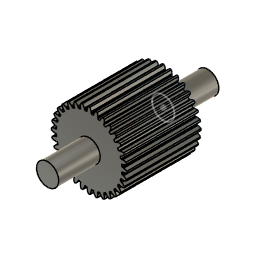
New_Spur_and_Rod v4 (Autodesk Fusion 360 design; units mm, degrees)
description: Spur Gear; Module: 0.750000; Number of Teeth: 32; Pressure Angle: 20.000000; Root Fillet Radius: 0.032000; Clearance: 0.000000; Gear Thickness: 2.500000; Hole Diameter: 0.750000;
Autodesk Fusion 360 part; units mm, degrees
sketch "Sketch1" plane through (0, 0, 0) normal (0, 1, 0) x (1, 0, 0) in component "Spur Gear (32 teeth)"
  arc A0 (10.9657, -1.4605) -> (11.0399, -0.7069) centre (0, 0) ccw
  line L0 (11.0399, -0.7069) -> (11.2693, -0.7216)
  spline S0 degree 3 poles (11.2693, -0.7216) (11.3119, -0.7221) (11.4405, -0.7189) (11.6548, -0.6748) knots 0 0 0 0 1 1 1 1
  spline S1 degree 3 poles (11.6548, -0.6748) (11.911, -0.6218) (12.2826, -0.5105) (12.7477, -0.2784) knots 0 0 0 0 1 1 1 1
  arc A1 (12.7477, -0.2784) -> (12.7477, 0.2784) centre (0, 0) ccw
  spline S2 degree 3 poles (12.7477, 0.2784) (12.2826, 0.5105) (11.911, 0.6218) (11.6548, 0.6748) knots 0 0 0 0 1 1 1 1
  spline S3 degree 3 poles (11.6548, 0.6748) (11.4405, 0.7189) (11.3119, 0.7221) (11.2693, 0.7216) knots 0 0 0 0 1 1 1 1
  line L1 (11.2693, 0.7216) -> (11.0399, 0.7069)
  arc A2 (11.0399, 0.7069) -> (10.9657, 1.4605) centre (0, 0) ccw
  line L2 (10.9657, 1.4605) -> (11.1935, 1.4908)
  spline S4 degree 3 poles (11.1935, 1.4908) (11.2354, 1.4987) (11.3609, 1.5268) (11.5625, 1.6119) knots 0 0 0 0 1 1 1 1
  spline S5 degree 3 poles (11.5625, 1.6119) (11.8034, 1.7139) (12.1462, 1.8956) (12.5571, 2.2139) knots 0 0 0 0 1 1 1 1
  arc A3 (12.5571, 2.2139) -> (12.4485, 2.76) centre (0, 0) ccw
  spline S6 degree 3 poles (12.4485, 2.76) (11.947, 2.8969) (11.5608, 2.9336) (11.2992, 2.9356) knots 0 0 0 0 1 1 1 1
  spline S7 degree 3 poles (11.2992, 2.9356) (11.0804, 2.937) (10.9537, 2.915) (10.912, 2.9063) knots 0 0 0 0 1 1 1 1
  line L3 (10.912, 2.9063) -> (10.6899, 2.8471)
  arc A4 (10.6899, 2.8471) -> (10.47, 3.5717) centre (0, 0) ccw
  line L4 (10.47, 3.5717) -> (10.6876, 3.6459)
  spline S8 degree 3 poles (10.6876, 3.6459) (10.7272, 3.6618) (10.8448, 3.7139) (11.0259, 3.8367) knots 0 0 0 0 1 1 1 1
  spline S9 degree 3 poles (11.0259, 3.8367) (11.2423, 3.9837) (11.543, 4.2287) (11.8839, 4.6211) knots 0 0 0 0 1 1 1 1
  arc A5 (11.8839, 4.6211) -> (11.6708, 5.1356) centre (0, 0) ccw
  spline S10 degree 3 poles (11.6708, 5.1356) (11.1523, 5.1719) (10.7664, 5.1326) (10.5094, 5.0835) knots 0 0 0 0 1 1 1 1
  spline S11 degree 3 poles (10.5094, 5.0835) (10.2945, 5.0423) (10.1746, 4.996) (10.1353, 4.9792) knots 0 0 0 0 1 1 1 1
  line L5 (10.1353, 4.9792) -> (9.929, 4.8779)
  arc A6 (9.929, 4.8779) -> (9.5721, 5.5457) centre (0, 0) ccw
  line L6 (9.5721, 5.5457) -> (9.771, 5.6609)
  spline S12 degree 3 poles (9.771, 5.6609) (9.8067, 5.6842) (9.9118, 5.7583) (10.0655, 5.914) knots 0 0 0 0 1 1 1 1
  spline S13 degree 3 poles (10.0655, 5.914) (10.2491, 6.1004) (10.4962, 6.3994) (10.754, 6.8508) knots 0 0 0 0 1 1 1 1
  arc A7 (10.754, 6.8508) -> (10.4447, 7.3137) centre (0, 0) ccw
  spline S14 degree 3 poles (10.4447, 7.3137) (9.929, 7.2483) (9.5582, 7.1344) (9.3157, 7.0361) knots 0 0 0 0 1 1 1 1
  spline S15 degree 3 poles (9.3157, 7.0361) (9.113, 6.9538) (9.0044, 6.8849) (8.9692, 6.8609) knots 0 0 0 0 1 1 1 1
  line L7 (8.9692, 6.8609) -> (8.7866, 6.7212)
  arc A8 (8.7866, 6.7212) -> (8.3062, 7.3065) centre (0, 0) ccw
  line L8 (8.3062, 7.3065) -> (8.4788, 7.4584)
  spline S16 degree 3 poles (8.4788, 7.4584) (8.5093, 7.4882) (8.598, 7.5813) (8.7184, 7.7641) knots 0 0 0 0 1 1 1 1
  spline S17 degree 3 poles (8.7184, 7.7641) (8.862, 7.9827) (9.046, 8.3242) (9.2109, 8.8171) knots 0 0 0 0 1 1 1 1
  arc A9 (9.2109, 8.8171) -> (8.8171, 9.2109) centre (0, 0) ccw
  spline S18 degree 3 poles (8.8171, 9.2109) (8.3242, 9.046) (7.9827, 8.862) (7.7641, 8.7184) knots 0 0 0 0 1 1 1 1
  spline S19 degree 3 poles (7.7641, 8.7184) (7.5813, 8.598) (7.4882, 8.5093) (7.4584, 8.4788) knots 0 0 0 0 1 1 1 1
  line L9 (7.4584, 8.4788) -> (7.3065, 8.3062)
  arc A10 (7.3065, 8.3062) -> (6.7212, 8.7866) centre (0, 0) ccw
  line L10 (6.7212, 8.7866) -> (6.8609, 8.9692)
  spline S20 degree 3 poles (6.8609, 8.9692) (6.8849, 9.0044) (6.9538, 9.113) (7.0361, 9.3157) knots 0 0 0 0 1 1 1 1
  spline S21 degree 3 poles (7.0361, 9.3157) (7.1344, 9.5582) (7.2483, 9.929) (7.3137, 10.4447) knots 0 0 0 0 1 1 1 1
  arc A11 (7.3137, 10.4447) -> (6.8508, 10.754) centre (0, 0) ccw
  spline S22 degree 3 poles (6.8508, 10.754) (6.3994, 10.4962) (6.1004, 10.2491) (5.914, 10.0655) knots 0 0 0 0 1 1 1 1
  spline S23 degree 3 poles (5.914, 10.0655) (5.7583, 9.9118) (5.6842, 9.8067) (5.6609, 9.771) knots 0 0 0 0 1 1 1 1
  line L11 (5.6609, 9.771) -> (5.5457, 9.5721)
  arc A12 (5.5457, 9.5721) -> (4.8779, 9.929) centre (0, 0) ccw
  line L12 (4.8779, 9.929) -> (4.9792, 10.1353)
  spline S24 degree 3 poles (4.9792, 10.1353) (4.996, 10.1746) (5.0423, 10.2945) (5.0835, 10.5094) knots 0 0 0 0 1 1 1 1
  spline S25 degree 3 poles (5.0835, 10.5094) (5.1326, 10.7664) (5.1719, 11.1523) (5.1356, 11.6708) knots 0 0 0 0 1 1 1 1
  arc A13 (5.1356, 11.6708) -> (4.6211, 11.8839) centre (0, 0) ccw
  spline S26 degree 3 poles (4.6211, 11.8839) (4.2287, 11.543) (3.9837, 11.2423) (3.8367, 11.0259) knots 0 0 0 0 1 1 1 1
  spline S27 degree 3 poles (3.8367, 11.0259) (3.7139, 10.8448) (3.6618, 10.7272) (3.6459, 10.6876) knots 0 0 0 0 1 1 1 1
  line L13 (3.6459, 10.6876) -> (3.5717, 10.47)
  arc A14 (3.5717, 10.47) -> (2.8471, 10.6899) centre (0, 0) ccw
  line L14 (2.8471, 10.6899) -> (2.9063, 10.912)
  spline S28 degree 3 poles (2.9063, 10.912) (2.915, 10.9537) (2.937, 11.0804) (2.9356, 11.2992) knots 0 0 0 0 1 1 1 1
  spline S29 degree 3 poles (2.9356, 11.2992) (2.9336, 11.5608) (2.8969, 11.947) (2.76, 12.4485) knots 0 0 0 0 1 1 1 1
  arc A15 (2.76, 12.4485) -> (2.2139, 12.5571) centre (0, 0) ccw
  spline S30 degree 3 poles (2.2139, 12.5571) (1.8956, 12.1462) (1.7139, 11.8034) (1.6119, 11.5625) knots 0 0 0 0 1 1 1 1
  spline S31 degree 3 poles (1.6119, 11.5625) (1.5268, 11.3609) (1.4987, 11.2354) (1.4908, 11.1935) knots 0 0 0 0 1 1 1 1
  line L15 (1.4908, 11.1935) -> (1.4605, 10.9657)
  arc A16 (1.4605, 10.9657) -> (0.7069, 11.0399) centre (0, 0) ccw
  line L16 (0.7069, 11.0399) -> (0.7216, 11.2693)
  spline S32 degree 3 poles (0.7216, 11.2693) (0.7221, 11.3119) (0.7189, 11.4405) (0.6748, 11.6548) knots 0 0 0 0 1 1 1 1
  spline S33 degree 3 poles (0.6748, 11.6548) (0.6218, 11.911) (0.5105, 12.2826) (0.2784, 12.7477) knots 0 0 0 0 1 1 1 1
  arc A17 (0.2784, 12.7477) -> (-0.2784, 12.7477) centre (0, 0) ccw
  spline S34 degree 3 poles (-0.2784, 12.7477) (-0.5105, 12.2826) (-0.6218, 11.911) (-0.6748, 11.6548) knots 0 0 0 0 1 1 1 1
  spline S35 degree 3 poles (-0.6748, 11.6548) (-0.7189, 11.4405) (-0.7221, 11.3119) (-0.7216, 11.2693) knots 0 0 0 0 1 1 1 1
  line L17 (-0.7216, 11.2693) -> (-0.7069, 11.0399)
  arc A18 (-0.7069, 11.0399) -> (-1.4605, 10.9657) centre (0, 0) ccw
  line L18 (-1.4605, 10.9657) -> (-1.4908, 11.1935)
  spline S36 degree 3 poles (-1.4908, 11.1935) (-1.4987, 11.2354) (-1.5268, 11.3609) (-1.6119, 11.5625) knots 0 0 0 0 1 1 1 1
  spline S37 degree 3 poles (-1.6119, 11.5625) (-1.7139, 11.8034) (-1.8956, 12.1462) (-2.2139, 12.5571) knots 0 0 0 0 1 1 1 1
  arc A19 (-2.2139, 12.5571) -> (-2.76, 12.4485) centre (0, 0) ccw
  spline S38 degree 3 poles (-2.76, 12.4485) (-2.8969, 11.947) (-2.9336, 11.5608) (-2.9356, 11.2992) knots 0 0 0 0 1 1 1 1
  spline S39 degree 3 poles (-2.9356, 11.2992) (-2.937, 11.0804) (-2.915, 10.9537) (-2.9063, 10.912) knots 0 0 0 0 1 1 1 1
  line L19 (-2.9063, 10.912) -> (-2.8471, 10.6899)
  arc A20 (-2.8471, 10.6899) -> (-3.5717, 10.47) centre (0, 0) ccw
  line L20 (-3.5717, 10.47) -> (-3.6459, 10.6876)
  spline S40 degree 3 poles (-3.6459, 10.6876) (-3.6618, 10.7272) (-3.7139, 10.8448) (-3.8367, 11.0259) knots 0 0 0 0 1 1 1 1
  spline S41 degree 3 poles (-3.8367, 11.0259) (-3.9837, 11.2423) (-4.2287, 11.543) (-4.6211, 11.8839) knots 0 0 0 0 1 1 1 1
  arc A21 (-4.6211, 11.8839) -> (-5.1356, 11.6708) centre (0, 0) ccw
  spline S42 degree 3 poles (-5.1356, 11.6708) (-5.1719, 11.1523) (-5.1326, 10.7664) (-5.0835, 10.5094) knots 0 0 0 0 1 1 1 1
  spline S43 degree 3 poles (-5.0835, 10.5094) (-5.0423, 10.2945) (-4.996, 10.1746) (-4.9792, 10.1353) knots 0 0 0 0 1 1 1 1
  line L21 (-4.9792, 10.1353) -> (-4.8779, 9.929)
  arc A22 (-4.8779, 9.929) -> (-5.5457, 9.5721) centre (0, 0) ccw
  line L22 (-5.5457, 9.5721) -> (-5.6609, 9.771)
  spline S44 degree 3 poles (-5.6609, 9.771) (-5.6842, 9.8067) (-5.7583, 9.9118) (-5.914, 10.0655) knots 0 0 0 0 1 1 1 1
  spline S45 degree 3 poles (-5.914, 10.0655) (-6.1004, 10.2491) (-6.3994, 10.4962) (-6.8508, 10.754) knots 0 0 0 0 1 1 1 1
  arc A23 (-6.8508, 10.754) -> (-7.3137, 10.4447) centre (0, 0) ccw
  spline S46 degree 3 poles (-7.3137, 10.4447) (-7.2483, 9.929) (-7.1344, 9.5582) (-7.0361, 9.3157) knots 0 0 0 0 1 1 1 1
  spline S47 degree 3 poles (-7.0361, 9.3157) (-6.9538, 9.113) (-6.8849, 9.0044) (-6.8609, 8.9692) knots 0 0 0 0 1 1 1 1
  line L23 (-6.8609, 8.9692) -> (-6.7212, 8.7866)
  arc A24 (-6.7212, 8.7866) -> (-7.3065, 8.3062) centre (0, 0) ccw
  line L24 (-7.3065, 8.3062) -> (-7.4584, 8.4788)
  spline S48 degree 3 poles (-7.4584, 8.4788) (-7.4882, 8.5093) (-7.5813, 8.598) (-7.7641, 8.7184) knots 0 0 0 0 1 1 1 1
  spline S49 degree 3 poles (-7.7641, 8.7184) (-7.9827, 8.862) (-8.3242, 9.046) (-8.8171, 9.2109) knots 0 0 0 0 1 1 1 1
  arc A25 (-8.8171, 9.2109) -> (-9.2109, 8.8171) centre (0, 0) ccw
  spline S50 degree 3 poles (-9.2109, 8.8171) (-9.046, 8.3242) (-8.862, 7.9827) (-8.7184, 7.7641) knots 0 0 0 0 1 1 1 1
  spline S51 degree 3 poles (-8.7184, 7.7641) (-8.598, 7.5813) (-8.5093, 7.4882) (-8.4788, 7.4584) knots 0 0 0 0 1 1 1 1
  line L25 (-8.4788, 7.4584) -> (-8.3062, 7.3065)
  arc A26 (-8.3062, 7.3065) -> (-8.7866, 6.7212) centre (0, 0) ccw
  line L26 (-8.7866, 6.7212) -> (-8.9692, 6.8609)
  spline S52 degree 3 poles (-8.9692, 6.8609) (-9.0044, 6.8849) (-9.113, 6.9538) (-9.3157, 7.0361) knots 0 0 0 0 1 1 1 1
  spline S53 degree 3 poles (-9.3157, 7.0361) (-9.5582, 7.1344) (-9.929, 7.2483) (-10.4447, 7.3137) knots 0 0 0 0 1 1 1 1
  arc A27 (-10.4447, 7.3137) -> (-10.754, 6.8508) centre (0, 0) ccw
  spline S54 degree 3 poles (-10.754, 6.8508) (-10.4962, 6.3994) (-10.2491, 6.1004) (-10.0655, 5.914) knots 0 0 0 0 1 1 1 1
  spline S55 degree 3 poles (-10.0655, 5.914) (-9.9118, 5.7583) (-9.8067, 5.6842) (-9.771, 5.6609) knots 0 0 0 0 1 1 1 1
  line L27 (-9.771, 5.6609) -> (-9.5721, 5.5457)
  arc A28 (-9.5721, 5.5457) -> (-9.929, 4.8779) centre (0, 0) ccw
  line L28 (-9.929, 4.8779) -> (-10.1353, 4.9792)
  spline S56 degree 3 poles (-10.1353, 4.9792) (-10.1746, 4.996) (-10.2945, 5.0423) (-10.5094, 5.0835) knots 0 0 0 0 1 1 1 1
  spline S57 degree 3 poles (-10.5094, 5.0835) (-10.7664, 5.1326) (-11.1523, 5.1719) (-11.6708, 5.1356) knots 0 0 0 0 1 1 1 1
  arc A29 (-11.6708, 5.1356) -> (-11.8839, 4.6211) centre (0, 0) ccw
  spline S58 degree 3 poles (-11.8839, 4.6211) (-11.543, 4.2287) (-11.2423, 3.9837) (-11.0259, 3.8367) knots 0 0 0 0 1 1 1 1
  spline S59 degree 3 poles (-11.0259, 3.8367) (-10.8448, 3.7139) (-10.7272, 3.6618) (-10.6876, 3.6459) knots 0 0 0 0 1 1 1 1
  line L29 (-10.6876, 3.6459) -> (-10.47, 3.5717)
  arc A30 (-10.47, 3.5717) -> (-10.6899, 2.8471) centre (0, 0) ccw
  line L30 (-10.6899, 2.8471) -> (-10.912, 2.9063)
  spline S60 degree 3 poles (-10.912, 2.9063) (-10.9537, 2.915) (-11.0804, 2.937) (-11.2992, 2.9356) knots 0 0 0 0 1 1 1 1
  spline S61 degree 3 poles (-11.2992, 2.9356) (-11.5608, 2.9336) (-11.947, 2.8969) (-12.4485, 2.76) knots 0 0 0 0 1 1 1 1
  arc A31 (-12.4485, 2.76) -> (-12.5571, 2.2139) centre (0, 0) ccw
  spline S62 degree 3 poles (-12.5571, 2.2139) (-12.1462, 1.8956) (-11.8034, 1.7139) (-11.5625, 1.6119) knots 0 0 0 0 1 1 1 1
  spline S63 degree 3 poles (-11.5625, 1.6119) (-11.3609, 1.5268) (-11.2354, 1.4987) (-11.1935, 1.4908) knots 0 0 0 0 1 1 1 1
  line L31 (-11.1935, 1.4908) -> (-10.9657, 1.4605)
  arc A32 (-10.9657, 1.4605) -> (-11.0399, 0.7069) centre (0, 0) ccw
  line L32 (-11.0399, 0.7069) -> (-11.2693, 0.7216)
  spline S64 degree 3 poles (-11.2693, 0.7216) (-11.3119, 0.7221) (-11.4405, 0.7189) (-11.6548, 0.6748) knots 0 0 0 0 1 1 1 1
  spline S65 degree 3 poles (-11.6548, 0.6748) (-11.911, 0.6218) (-12.2826, 0.5105) (-12.7477, 0.2784) knots 0 0 0 0 1 1 1 1
  arc A33 (-12.7477, 0.2784) -> (-12.7477, -0.2784) centre (0, 0) ccw
  spline S66 degree 3 poles (-12.7477, -0.2784) (-12.2826, -0.5105) (-11.911, -0.6218) (-11.6548, -0.6748) knots 0 0 0 0 1 1 1 1
  spline S67 degree 3 poles (-11.6548, -0.6748) (-11.4405, -0.7189) (-11.3119, -0.7221) (-11.2693, -0.7216) knots 0 0 0 0 1 1 1 1
  line L33 (-11.2693, -0.7216) -> (-11.0399, -0.7069)
  arc A34 (-11.0399, -0.7069) -> (-10.9657, -1.4605) centre (0, 0) ccw
  line L34 (-10.9657, -1.4605) -> (-11.1935, -1.4908)
  spline S68 degree 3 poles (-11.1935, -1.4908) (-11.2354, -1.4987) (-11.3609, -1.5268) (-11.5625, -1.6119) knots 0 0 0 0 1 1 1 1
  spline S69 degree 3 poles (-11.5625, -1.6119) (-11.8034, -1.7139) (-12.1462, -1.8956) (-12.5571, -2.2139) knots 0 0 0 0 1 1 1 1
  arc A35 (-12.5571, -2.2139) -> (-12.4485, -2.76) centre (0, 0) ccw
  spline S70 degree 3 poles (-12.4485, -2.76) (-11.947, -2.8969) (-11.5608, -2.9336) (-11.2992, -2.9356) knots 0 0 0 0 1 1 1 1
  spline S71 degree 3 poles (-11.2992, -2.9356) (-11.0804, -2.937) (-10.9537, -2.915) (-10.912, -2.9063) knots 0 0 0 0 1 1 1 1
  line L35 (-10.912, -2.9063) -> (-10.6899, -2.8471)
  arc A36 (-10.6899, -2.8471) -> (-10.47, -3.5717) centre (0, 0) ccw
  line L36 (-10.47, -3.5717) -> (-10.6876, -3.6459)
  spline S72 degree 3 poles (-10.6876, -3.6459) (-10.7272, -3.6618) (-10.8448, -3.7139) (-11.0259, -3.8367) knots 0 0 0 0 1 1 1 1
  spline S73 degree 3 poles (-11.0259, -3.8367) (-11.2423, -3.9837) (-11.543, -4.2287) (-11.8839, -4.6211) knots 0 0 0 0 1 1 1 1
  arc A37 (-11.8839, -4.6211) -> (-11.6708, -5.1356) centre (0, 0) ccw
  spline S74 degree 3 poles (-11.6708, -5.1356) (-11.1523, -5.1719) (-10.7664, -5.1326) (-10.5094, -5.0835) knots 0 0 0 0 1 1 1 1
  spline S75 degree 3 poles (-10.5094, -5.0835) (-10.2945, -5.0423) (-10.1746, -4.996) (-10.1353, -4.9792) knots 0 0 0 0 1 1 1 1
  line L37 (-10.1353, -4.9792) -> (-9.929, -4.8779)
  arc A38 (-9.929, -4.8779) -> (-9.5721, -5.5457) centre (0, 0) ccw
  line L38 (-9.5721, -5.5457) -> (-9.771, -5.6609)
  spline S76 degree 3 poles (-9.771, -5.6609) (-9.8067, -5.6842) (-9.9118, -5.7583) (-10.0655, -5.914) knots 0 0 0 0 1 1 1 1
  spline S77 degree 3 poles (-10.0655, -5.914) (-10.2491, -6.1004) (-10.4962, -6.3994) (-10.754, -6.8508) knots 0 0 0 0 1 1 1 1
  arc A39 (-10.754, -6.8508) -> (-10.4447, -7.3137) centre (0, 0) ccw
  spline S78 degree 3 poles (-10.4447, -7.3137) (-9.929, -7.2483) (-9.5582, -7.1344) (-9.3157, -7.0361) knots 0 0 0 0 1 1 1 1
  spline S79 degree 3 poles (-9.3157, -7.0361) (-9.113, -6.9538) (-9.0044, -6.8849) (-8.9692, -6.8609) knots 0 0 0 0 1 1 1 1
  line L39 (-8.9692, -6.8609) -> (-8.7866, -6.7212)
  arc A40 (-8.7866, -6.7212) -> (-8.3062, -7.3065) centre (0, 0) ccw
  line L40 (-8.3062, -7.3065) -> (-8.4788, -7.4584)
  spline S80 degree 3 poles (-8.4788, -7.4584) (-8.5093, -7.4882) (-8.598, -7.5813) (-8.7184, -7.7641) knots 0 0 0 0 1 1 1 1
  spline S81 degree 3 poles (-8.7184, -7.7641) (-8.862, -7.9827) (-9.046, -8.3242) (-9.2109, -8.8171) knots 0 0 0 0 1 1 1 1
  arc A41 (-9.2109, -8.8171) -> (-8.8171, -9.2109) centre (0, 0) ccw
  spline S82 degree 3 poles (-8.8171, -9.2109) (-8.3242, -9.046) (-7.9827, -8.862) (-7.7641, -8.7184) knots 0 0 0 0 1 1 1 1
  spline S83 degree 3 poles (-7.7641, -8.7184) (-7.5813, -8.598) (-7.4882, -8.5093) (-7.4584, -8.4788) knots 0 0 0 0 1 1 1 1
  line L41 (-7.4584, -8.4788) -> (-7.3065, -8.3062)
  arc A42 (-7.3065, -8.3062) -> (-6.7212, -8.7866) centre (0, 0) ccw
  line L42 (-6.7212, -8.7866) -> (-6.8609, -8.9692)
  spline S84 degree 3 poles (-6.8609, -8.9692) (-6.8849, -9.0044) (-6.9538, -9.113) (-7.0361, -9.3157) knots 0 0 0 0 1 1 1 1
  spline S85 degree 3 poles (-7.0361, -9.3157) (-7.1344, -9.5582) (-7.2483, -9.929) (-7.3137, -10.4447) knots 0 0 0 0 1 1 1 1
  arc A43 (-7.3137, -10.4447) -> (-6.8508, -10.754) centre (0, 0) ccw
  spline S86 degree 3 poles (-6.8508, -10.754) (-6.3994, -10.4962) (-6.1004, -10.2491) (-5.914, -10.0655) knots 0 0 0 0 1 1 1 1
  spline S87 degree 3 poles (-5.914, -10.0655) (-5.7583, -9.9118) (-5.6842, -9.8067) (-5.6609, -9.771) knots 0 0 0 0 1 1 1 1
  line L43 (-5.6609, -9.771) -> (-5.5457, -9.5721)
  arc A44 (-5.5457, -9.5721) -> (-4.8779, -9.929) centre (0, 0) ccw
  line L44 (-4.8779, -9.929) -> (-4.9792, -10.1353)
  spline S88 degree 3 poles (-4.9792, -10.1353) (-4.996, -10.1746) (-5.0423, -10.2945) (-5.0835, -10.5094) knots 0 0 0 0 1 1 1 1
  spline S89 degree 3 poles (-5.0835, -10.5094) (-5.1326, -10.7664) (-5.1719, -11.1523) (-5.1356, -11.6708) knots 0 0 0 0 1 1 1 1
  arc A45 (-5.1356, -11.6708) -> (-4.6211, -11.8839) centre (0, 0) ccw
  spline S90 degree 3 poles (-4.6211, -11.8839) (-4.2287, -11.543) (-3.9837, -11.2423) (-3.8367, -11.0259) knots 0 0 0 0 1 1 1 1
  spline S91 degree 3 poles (-3.8367, -11.0259) (-3.7139, -10.8448) (-3.6618, -10.7272) (-3.6459, -10.6876) knots 0 0 0 0 1 1 1 1
  line L45 (-3.6459, -10.6876) -> (-3.5717, -10.47)
  arc A46 (-3.5717, -10.47) -> (-2.8471, -10.6899) centre (0, 0) ccw
  line L46 (-2.8471, -10.6899) -> (-2.9063, -10.912)
  spline S92 degree 3 poles (-2.9063, -10.912) (-2.915, -10.9537) (-2.937, -11.0804) (-2.9356, -11.2992) knots 0 0 0 0 1 1 1 1
  spline S93 degree 3 poles (-2.9356, -11.2992) (-2.9336, -11.5608) (-2.8969, -11.947) (-2.76, -12.4485) knots 0 0 0 0 1 1 1 1
  arc A47 (-2.76, -12.4485) -> (-2.2139, -12.5571) centre (0, 0) ccw
  spline S94 degree 3 poles (-2.2139, -12.5571) (-1.8956, -12.1462) (-1.7139, -11.8034) (-1.6119, -11.5625) knots 0 0 0 0 1 1 1 1
  spline S95 degree 3 poles (-1.6119, -11.5625) (-1.5268, -11.3609) (-1.4987, -11.2354) (-1.4908, -11.1935) knots 0 0 0 0 1 1 1 1
  line L47 (-1.4908, -11.1935) -> (-1.4605, -10.9657)
  arc A48 (-1.4605, -10.9657) -> (-0.7069, -11.0399) centre (0, 0) ccw
  line L48 (-0.7069, -11.0399) -> (-0.7216, -11.2693)
  spline S96 degree 3 poles (-0.7216, -11.2693) (-0.7221, -11.3119) (-0.7189, -11.4405) (-0.6748, -11.6548) knots 0 0 0 0 1 1 1 1
  spline S97 degree 3 poles (-0.6748, -11.6548) (-0.6218, -11.911) (-0.5105, -12.2826) (-0.2784, -12.7477) knots 0 0 0 0 1 1 1 1
  arc A49 (-0.2784, -12.7477) -> (0.2784, -12.7477) centre (0, 0) ccw
  spline S98 degree 3 poles (0.2784, -12.7477) (0.5105, -12.2826) (0.6218, -11.911) (0.6748, -11.6548) knots 0 0 0 0 1 1 1 1
  spline S99 degree 3 poles (0.6748, -11.6548) (0.7189, -11.4405) (0.7221, -11.3119) (0.7216, -11.2693) knots 0 0 0 0 1 1 1 1
  line L49 (0.7216, -11.2693) -> (0.7069, -11.0399)
  arc A50 (0.7069, -11.0399) -> (1.4605, -10.9657) centre (0, 0) ccw
  line L50 (1.4605, -10.9657) -> (1.4908, -11.1935)
  spline S100 degree 3 poles (1.4908, -11.1935) (1.4987, -11.2354) (1.5268, -11.3609) (1.6119, -11.5625) knots 0 0 0 0 1 1 1 1
  spline S101 degree 3 poles (1.6119, -11.5625) (1.7139, -11.8034) (1.8956, -12.1462) (2.2139, -12.5571) knots 0 0 0 0 1 1 1 1
  arc A51 (2.2139, -12.5571) -> (2.76, -12.4485) centre (0, 0) ccw
  spline S102 degree 3 poles (2.76, -12.4485) (2.8969, -11.947) (2.9336, -11.5608) (2.9356, -11.2992) knots 0 0 0 0 1 1 1 1
  spline S103 degree 3 poles (2.9356, -11.2992) (2.937, -11.0804) (2.915, -10.9537) (2.9063, -10.912) knots 0 0 0 0 1 1 1 1
  line L51 (2.9063, -10.912) -> (2.8471, -10.6899)
  arc A52 (2.8471, -10.6899) -> (3.5717, -10.47) centre (0, 0) ccw
  line L52 (3.5717, -10.47) -> (3.6459, -10.6876)
  spline S104 degree 3 poles (3.6459, -10.6876) (3.6618, -10.7272) (3.7139, -10.8448) (3.8367, -11.0259) knots 0 0 0 0 1 1 1 1
  spline S105 degree 3 poles (3.8367, -11.0259) (3.9837, -11.2423) (4.2287, -11.543) (4.6211, -11.8839) knots 0 0 0 0 1 1 1 1
  arc A53 (4.6211, -11.8839) -> (5.1356, -11.6708) centre (0, 0) ccw
  spline S106 degree 3 poles (5.1356, -11.6708) (5.1719, -11.1523) (5.1326, -10.7664) (5.0835, -10.5094) knots 0 0 0 0 1 1 1 1
  spline S107 degree 3 poles (5.0835, -10.5094) (5.0423, -10.2945) (4.996, -10.1746) (4.9792, -10.1353) knots 0 0 0 0 1 1 1 1
  line L53 (4.9792, -10.1353) -> (4.8779, -9.929)
  arc A54 (4.8779, -9.929) -> (5.5457, -9.5721) centre (0, 0) ccw
  line L54 (5.5457, -9.5721) -> (5.6609, -9.771)
  spline S108 degree 3 poles (5.6609, -9.771) (5.6842, -9.8067) (5.7583, -9.9118) (5.914, -10.0655) knots 0 0 0 0 1 1 1 1
  spline S109 degree 3 poles (5.914, -10.0655) (6.1004, -10.2491) (6.3994, -10.4962) (6.8508, -10.754) knots 0 0 0 0 1 1 1 1
  arc A55 (6.8508, -10.754) -> (7.3137, -10.4447) centre (0, 0) ccw
  spline S110 degree 3 poles (7.3137, -10.4447) (7.2483, -9.929) (7.1344, -9.5582) (7.0361, -9.3157) knots 0 0 0 0 1 1 1 1
  spline S111 degree 3 poles (7.0361, -9.3157) (6.9538, -9.113) (6.8849, -9.0044) (6.8609, -8.9692) knots 0 0 0 0 1 1 1 1
  line L55 (6.8609, -8.9692) -> (6.7212, -8.7866)
  arc A56 (6.7212, -8.7866) -> (7.3065, -8.3062) centre (0, 0) ccw
  line L56 (7.3065, -8.3062) -> (7.4584, -8.4788)
  spline S112 degree 3 poles (7.4584, -8.4788) (7.4882, -8.5093) (7.5813, -8.598) (7.7641, -8.7184) knots 0 0 0 0 1 1 1 1
  spline S113 degree 3 poles (7.7641, -8.7184) (7.9827, -8.862) (8.3242, -9.046) (8.8171, -9.2109) knots 0 0 0 0 1 1 1 1
  arc A57 (8.8171, -9.2109) -> (9.2109, -8.8171) centre (0, 0) ccw
  spline S114 degree 3 poles (9.2109, -8.8171) (9.046, -8.3242) (8.862, -7.9827) (8.7184, -7.7641) knots 0 0 0 0 1 1 1 1
  spline S115 degree 3 poles (8.7184, -7.7641) (8.598, -7.5813) (8.5093, -7.4882) (8.4788, -7.4584) knots 0 0 0 0 1 1 1 1
  line L57 (8.4788, -7.4584) -> (8.3062, -7.3065)
  arc A58 (8.3062, -7.3065) -> (8.7866, -6.7212) centre (0, 0) ccw
  line L58 (8.7866, -6.7212) -> (8.9692, -6.8609)
  spline S116 degree 3 poles (8.9692, -6.8609) (9.0044, -6.8849) (9.113, -6.9538) (9.3157, -7.0361) knots 0 0 0 0 1 1 1 1
  spline S117 degree 3 poles (9.3157, -7.0361) (9.5582, -7.1344) (9.929, -7.2483) (10.4447, -7.3137) knots 0 0 0 0 1 1 1 1
  arc A59 (10.4447, -7.3137) -> (10.754, -6.8508) centre (0, 0) ccw
  spline S118 degree 3 poles (10.754, -6.8508) (10.4962, -6.3994) (10.2491, -6.1004) (10.0655, -5.914) knots 0 0 0 0 1 1 1 1
  spline S119 degree 3 poles (10.0655, -5.914) (9.9118, -5.7583) (9.8067, -5.6842) (9.771, -5.6609) knots 0 0 0 0 1 1 1 1
  line L59 (9.771, -5.6609) -> (9.5721, -5.5457)
  arc A60 (9.5721, -5.5457) -> (9.929, -4.8779) centre (0, 0) ccw
  line L60 (9.929, -4.8779) -> (10.1353, -4.9792)
  spline S120 degree 3 poles (10.1353, -4.9792) (10.1746, -4.996) (10.2945, -5.0423) (10.5094, -5.0835) knots 0 0 0 0 1 1 1 1
  spline S121 degree 3 poles (10.5094, -5.0835) (10.7664, -5.1326) (11.1523, -5.1719) (11.6708, -5.1356) knots 0 0 0 0 1 1 1 1
  arc A61 (11.6708, -5.1356) -> (11.8839, -4.6211) centre (0, 0) ccw
  spline S122 degree 3 poles (11.8839, -4.6211) (11.543, -4.2287) (11.2423, -3.9837) (11.0259, -3.8367) knots 0 0 0 0 1 1 1 1
  spline S123 degree 3 poles (11.0259, -3.8367) (10.8448, -3.7139) (10.7272, -3.6618) (10.6876, -3.6459) knots 0 0 0 0 1 1 1 1
  line L61 (10.6876, -3.6459) -> (10.47, -3.5717)
  arc A62 (10.47, -3.5717) -> (10.6899, -2.8471) centre (0, 0) ccw
  line L62 (10.6899, -2.8471) -> (10.912, -2.9063)
  spline S124 degree 3 poles (10.912, -2.9063) (10.9537, -2.915) (11.0804, -2.937) (11.2992, -2.9356) knots 0 0 0 0 1 1 1 1
  spline S125 degree 3 poles (11.2992, -2.9356) (11.5608, -2.9336) (11.947, -2.8969) (12.4485, -2.76) knots 0 0 0 0 1 1 1 1
  arc A63 (12.4485, -2.76) -> (12.5571, -2.2139) centre (0, 0) ccw
  spline S126 degree 3 poles (12.5571, -2.2139) (12.1462, -1.8956) (11.8034, -1.7139) (11.5625, -1.6119) knots 0 0 0 0 1 1 1 1
  spline S127 degree 3 poles (11.5625, -1.6119) (11.3609, -1.5268) (11.2354, -1.4987) (11.1935, -1.4908) knots 0 0 0 0 1 1 1 1
  line L63 (11.1935, -1.4908) -> (10.9657, -1.4605)
  circle A64 centre (0, 0) radius 3.75
extrude "Extrude1" add sketch "Sketch1" along normal blind 25 in component "Spur Gear (32 teeth)"
sketch "Sketch2" plane through (0, 0, 0) normal (0, 1, 0) x (1, 0, 0) in component "Spur Gear (32 teeth)"
  circle A0 centre (0, 0) radius 12 construction
sketch "Sketch1 (2)" plane through (0, 25, 0) normal (0, 1, 0) x (-1, 0, 0)
  circle A0 centre (0, 0) radius 3.75
  line L0 (-11.1935, 1.4908) -> (-10.9657, 1.4605)
  arc A1 (-10.9657, 1.4605) -> (-11.0399, 0.7069) centre (0, 0) ccw
  line L1 (-11.0399, 0.7069) -> (-11.2693, 0.7216)
  spline S0 degree 3 poles (-11.2693, 0.7216) (-11.3119, 0.7221) (-11.4405, 0.7189) (-11.6548, 0.6748) knots 0 0 0 0 1 1 1 1
  spline S1 degree 3 poles (-11.6548, 0.6748) (-11.911, 0.6218) (-12.2826, 0.5105) (-12.7477, 0.2784) knots 0 0 0 0 1 1 1 1
  arc A2 (-12.7477, 0.2784) -> (-12.7477, -0.2784) centre (0, 0) ccw
  spline S2 degree 3 poles (-12.7477, -0.2784) (-12.2826, -0.5105) (-11.911, -0.6218) (-11.6548, -0.6748) knots 0 0 0 0 1 1 1 1
  spline S3 degree 3 poles (-11.6548, -0.6748) (-11.4405, -0.7189) (-11.3119, -0.7221) (-11.2693, -0.7216) knots 0 0 0 0 1 1 1 1
  line L2 (-11.2693, -0.7216) -> (-11.0399, -0.7069)
  arc A3 (-11.0399, -0.7069) -> (-10.9657, -1.4605) centre (0, 0) ccw
  line L3 (-10.9657, -1.4605) -> (-11.1935, -1.4908)
  spline S4 degree 3 poles (-11.1935, -1.4908) (-11.2354, -1.4987) (-11.3609, -1.5268) (-11.5625, -1.6119) knots 0 0 0 0 1 1 1 1
  spline S5 degree 3 poles (-11.5625, -1.6119) (-11.8034, -1.7139) (-12.1462, -1.8956) (-12.5571, -2.2139) knots 0 0 0 0 1 1 1 1
  arc A4 (-12.5571, -2.2139) -> (-12.4485, -2.76) centre (0, 0) ccw
  spline S6 degree 3 poles (-12.4485, -2.76) (-11.947, -2.8969) (-11.5608, -2.9336) (-11.2992, -2.9356) knots 0 0 0 0 1 1 1 1
  spline S7 degree 3 poles (-11.2992, -2.9356) (-11.0804, -2.937) (-10.9537, -2.915) (-10.912, -2.9063) knots 0 0 0 0 1 1 1 1
  line L4 (-10.912, -2.9063) -> (-10.6899, -2.8471)
  arc A5 (-10.6899, -2.8471) -> (-10.47, -3.5717) centre (0, 0) ccw
  line L5 (-10.47, -3.5717) -> (-10.6876, -3.6459)
  spline S8 degree 3 poles (-10.6876, -3.6459) (-10.7272, -3.6618) (-10.8448, -3.7139) (-11.0259, -3.8367) knots 0 0 0 0 1 1 1 1
  spline S9 degree 3 poles (-11.0259, -3.8367) (-11.2423, -3.9837) (-11.543, -4.2287) (-11.8839, -4.6211) knots 0 0 0 0 1 1 1 1
  arc A6 (-11.8839, -4.6211) -> (-11.6708, -5.1356) centre (0, 0) ccw
  spline S10 degree 3 poles (-11.6708, -5.1356) (-11.1523, -5.1719) (-10.7664, -5.1326) (-10.5094, -5.0835) knots 0 0 0 0 1 1 1 1
  spline S11 degree 3 poles (-10.5094, -5.0835) (-10.2945, -5.0423) (-10.1746, -4.996) (-10.1353, -4.9792) knots 0 0 0 0 1 1 1 1
  line L6 (-10.1353, -4.9792) -> (-9.929, -4.8779)
  arc A7 (-9.929, -4.8779) -> (-9.5721, -5.5457) centre (0, 0) ccw
  line L7 (-9.5721, -5.5457) -> (-9.771, -5.6609)
  spline S12 degree 3 poles (-9.771, -5.6609) (-9.8067, -5.6842) (-9.9118, -5.7583) (-10.0655, -5.914) knots 0 0 0 0 1 1 1 1
  spline S13 degree 3 poles (-10.0655, -5.914) (-10.2491, -6.1004) (-10.4962, -6.3994) (-10.754, -6.8508) knots 0 0 0 0 1 1 1 1
  arc A8 (-10.754, -6.8508) -> (-10.4447, -7.3137) centre (0, 0) ccw
  spline S14 degree 3 poles (-10.4447, -7.3137) (-9.929, -7.2483) (-9.5582, -7.1344) (-9.3157, -7.0361) knots 0 0 0 0 1 1 1 1
  spline S15 degree 3 poles (-9.3157, -7.0361) (-9.113, -6.9538) (-9.0044, -6.8849) (-8.9692, -6.8609) knots 0 0 0 0 1 1 1 1
  line L8 (-8.9692, -6.8609) -> (-8.7866, -6.7212)
  arc A9 (-8.7866, -6.7212) -> (-8.3062, -7.3065) centre (0, 0) ccw
  line L9 (-8.3062, -7.3065) -> (-8.4788, -7.4584)
  spline S16 degree 3 poles (-8.4788, -7.4584) (-8.5093, -7.4882) (-8.598, -7.5813) (-8.7184, -7.7641) knots 0 0 0 0 1 1 1 1
  spline S17 degree 3 poles (-8.7184, -7.7641) (-8.862, -7.9827) (-9.046, -8.3242) (-9.2109, -8.8171) knots 0 0 0 0 1 1 1 1
  arc A10 (-9.2109, -8.8171) -> (-8.8171, -9.2109) centre (0, 0) ccw
  spline S18 degree 3 poles (-8.8171, -9.2109) (-8.3242, -9.046) (-7.9827, -8.862) (-7.7641, -8.7184) knots 0 0 0 0 1 1 1 1
  spline S19 degree 3 poles (-7.7641, -8.7184) (-7.5813, -8.598) (-7.4882, -8.5093) (-7.4584, -8.4788) knots 0 0 0 0 1 1 1 1
  line L10 (-7.4584, -8.4788) -> (-7.3065, -8.3062)
  arc A11 (-7.3065, -8.3062) -> (-6.7212, -8.7866) centre (0, 0) ccw
  line L11 (-6.7212, -8.7866) -> (-6.8609, -8.9692)
  spline S20 degree 3 poles (-6.8609, -8.9692) (-6.8849, -9.0044) (-6.9538, -9.113) (-7.0361, -9.3157) knots 0 0 0 0 1 1 1 1
  spline S21 degree 3 poles (-7.0361, -9.3157) (-7.1344, -9.5582) (-7.2483, -9.929) (-7.3137, -10.4447) knots 0 0 0 0 1 1 1 1
  arc A12 (-7.3137, -10.4447) -> (-6.8508, -10.754) centre (0, 0) ccw
  spline S22 degree 3 poles (-6.8508, -10.754) (-6.3994, -10.4962) (-6.1004, -10.2491) (-5.914, -10.0655) knots 0 0 0 0 1 1 1 1
  spline S23 degree 3 poles (-5.914, -10.0655) (-5.7583, -9.9118) (-5.6842, -9.8067) (-5.6609, -9.771) knots 0 0 0 0 1 1 1 1
  line L12 (-5.6609, -9.771) -> (-5.5457, -9.5721)
  arc A13 (-5.5457, -9.5721) -> (-4.8779, -9.929) centre (0, 0) ccw
  line L13 (-4.8779, -9.929) -> (-4.9792, -10.1353)
  spline S24 degree 3 poles (-4.9792, -10.1353) (-4.996, -10.1746) (-5.0423, -10.2945) (-5.0835, -10.5094) knots 0 0 0 0 1 1 1 1
  spline S25 degree 3 poles (-5.0835, -10.5094) (-5.1326, -10.7664) (-5.1719, -11.1523) (-5.1356, -11.6708) knots 0 0 0 0 1 1 1 1
  arc A14 (-5.1356, -11.6708) -> (-4.6211, -11.8839) centre (0, 0) ccw
  spline S26 degree 3 poles (-4.6211, -11.8839) (-4.2287, -11.543) (-3.9837, -11.2423) (-3.8367, -11.0259) knots 0 0 0 0 1 1 1 1
  spline S27 degree 3 poles (-3.8367, -11.0259) (-3.7139, -10.8448) (-3.6618, -10.7272) (-3.6459, -10.6876) knots 0 0 0 0 1 1 1 1
  line L14 (-3.6459, -10.6876) -> (-3.5717, -10.47)
  arc A15 (-3.5717, -10.47) -> (-2.8471, -10.6899) centre (0, 0) ccw
  line L15 (-2.8471, -10.6899) -> (-2.9063, -10.912)
  spline S28 degree 3 poles (-2.9063, -10.912) (-2.915, -10.9537) (-2.937, -11.0804) (-2.9356, -11.2992) knots 0 0 0 0 1 1 1 1
  spline S29 degree 3 poles (-2.9356, -11.2992) (-2.9336, -11.5608) (-2.8969, -11.947) (-2.76, -12.4485) knots 0 0 0 0 1 1 1 1
  arc A16 (-2.76, -12.4485) -> (-2.2139, -12.5571) centre (0, 0) ccw
  spline S30 degree 3 poles (-2.2139, -12.5571) (-1.8956, -12.1462) (-1.7139, -11.8034) (-1.6119, -11.5625) knots 0 0 0 0 1 1 1 1
  spline S31 degree 3 poles (-1.6119, -11.5625) (-1.5268, -11.3609) (-1.4987, -11.2354) (-1.4908, -11.1935) knots 0 0 0 0 1 1 1 1
  line L16 (-1.4908, -11.1935) -> (-1.4605, -10.9657)
  arc A17 (-1.4605, -10.9657) -> (-0.7069, -11.0399) centre (0, 0) ccw
  line L17 (-0.7069, -11.0399) -> (-0.7216, -11.2693)
  spline S32 degree 3 poles (-0.7216, -11.2693) (-0.7221, -11.3119) (-0.7189, -11.4405) (-0.6748, -11.6548) knots 0 0 0 0 1 1 1 1
  spline S33 degree 3 poles (-0.6748, -11.6548) (-0.6218, -11.911) (-0.5105, -12.2826) (-0.2784, -12.7477) knots 0 0 0 0 1 1 1 1
  arc A18 (-0.2784, -12.7477) -> (0.2784, -12.7477) centre (0, 0) ccw
  spline S34 degree 3 poles (0.2784, -12.7477) (0.5105, -12.2826) (0.6218, -11.911) (0.6748, -11.6548) knots 0 0 0 0 1 1 1 1
  spline S35 degree 3 poles (0.6748, -11.6548) (0.7189, -11.4405) (0.7221, -11.3119) (0.7216, -11.2693) knots 0 0 0 0 1 1 1 1
  line L18 (0.7216, -11.2693) -> (0.7069, -11.0399)
  arc A19 (0.7069, -11.0399) -> (1.4605, -10.9657) centre (0, 0) ccw
  line L19 (1.4605, -10.9657) -> (1.4908, -11.1935)
  spline S36 degree 3 poles (1.4908, -11.1935) (1.4987, -11.2354) (1.5268, -11.3609) (1.6119, -11.5625) knots 0 0 0 0 1 1 1 1
  spline S37 degree 3 poles (1.6119, -11.5625) (1.7139, -11.8034) (1.8956, -12.1462) (2.2139, -12.5571) knots 0 0 0 0 1 1 1 1
  arc A20 (2.2139, -12.5571) -> (2.76, -12.4485) centre (0, 0) ccw
  spline S38 degree 3 poles (2.76, -12.4485) (2.8969, -11.947) (2.9336, -11.5608) (2.9356, -11.2992) knots 0 0 0 0 1 1 1 1
  spline S39 degree 3 poles (2.9356, -11.2992) (2.937, -11.0804) (2.915, -10.9537) (2.9063, -10.912) knots 0 0 0 0 1 1 1 1
  line L20 (2.9063, -10.912) -> (2.8471, -10.6899)
  arc A21 (2.8471, -10.6899) -> (3.5717, -10.47) centre (0, 0) ccw
  line L21 (3.5717, -10.47) -> (3.6459, -10.6876)
  spline S40 degree 3 poles (3.6459, -10.6876) (3.6618, -10.7272) (3.7139, -10.8448) (3.8367, -11.0259) knots 0 0 0 0 1 1 1 1
  spline S41 degree 3 poles (3.8367, -11.0259) (3.9837, -11.2423) (4.2287, -11.543) (4.6211, -11.8839) knots 0 0 0 0 1 1 1 1
  arc A22 (4.6211, -11.8839) -> (5.1356, -11.6708) centre (0, 0) ccw
  spline S42 degree 3 poles (5.1356, -11.6708) (5.1719, -11.1523) (5.1326, -10.7664) (5.0835, -10.5094) knots 0 0 0 0 1 1 1 1
  spline S43 degree 3 poles (5.0835, -10.5094) (5.0423, -10.2945) (4.996, -10.1746) (4.9792, -10.1353) knots 0 0 0 0 1 1 1 1
  line L22 (4.9792, -10.1353) -> (4.8779, -9.929)
  arc A23 (4.8779, -9.929) -> (5.5457, -9.5721) centre (0, 0) ccw
  line L23 (5.5457, -9.5721) -> (5.6609, -9.771)
  spline S44 degree 3 poles (5.6609, -9.771) (5.6842, -9.8067) (5.7583, -9.9118) (5.914, -10.0655) knots 0 0 0 0 1 1 1 1
  spline S45 degree 3 poles (5.914, -10.0655) (6.1004, -10.2491) (6.3994, -10.4962) (6.8508, -10.754) knots 0 0 0 0 1 1 1 1
  arc A24 (6.8508, -10.754) -> (7.3137, -10.4447) centre (0, 0) ccw
  spline S46 degree 3 poles (7.3137, -10.4447) (7.2483, -9.929) (7.1344, -9.5582) (7.0361, -9.3157) knots 0 0 0 0 1 1 1 1
  spline S47 degree 3 poles (7.0361, -9.3157) (6.9538, -9.113) (6.8849, -9.0044) (6.8609, -8.9692) knots 0 0 0 0 1 1 1 1
  line L24 (6.8609, -8.9692) -> (6.7212, -8.7866)
  arc A25 (6.7212, -8.7866) -> (7.3065, -8.3062) centre (0, 0) ccw
  line L25 (7.3065, -8.3062) -> (7.4584, -8.4788)
  spline S48 degree 3 poles (7.4584, -8.4788) (7.4882, -8.5093) (7.5813, -8.598) (7.7641, -8.7184) knots 0 0 0 0 1 1 1 1
  spline S49 degree 3 poles (7.7641, -8.7184) (7.9827, -8.862) (8.3242, -9.046) (8.8171, -9.2109) knots 0 0 0 0 1 1 1 1
  arc A26 (8.8171, -9.2109) -> (9.2109, -8.8171) centre (0, 0) ccw
  spline S50 degree 3 poles (9.2109, -8.8171) (9.046, -8.3242) (8.862, -7.9827) (8.7184, -7.7641) knots 0 0 0 0 1 1 1 1
  spline S51 degree 3 poles (8.7184, -7.7641) (8.598, -7.5813) (8.5093, -7.4882) (8.4788, -7.4584) knots 0 0 0 0 1 1 1 1
  line L26 (8.4788, -7.4584) -> (8.3062, -7.3065)
  arc A27 (8.3062, -7.3065) -> (8.7866, -6.7212) centre (0, 0) ccw
  line L27 (8.7866, -6.7212) -> (8.9692, -6.8609)
  spline S52 degree 3 poles (8.9692, -6.8609) (9.0044, -6.8849) (9.113, -6.9538) (9.3157, -7.0361) knots 0 0 0 0 1 1 1 1
  spline S53 degree 3 poles (9.3157, -7.0361) (9.5582, -7.1344) (9.929, -7.2483) (10.4447, -7.3137) knots 0 0 0 0 1 1 1 1
  arc A28 (10.4447, -7.3137) -> (10.754, -6.8508) centre (0, 0) ccw
  spline S54 degree 3 poles (10.754, -6.8508) (10.4962, -6.3994) (10.2491, -6.1004) (10.0655, -5.914) knots 0 0 0 0 1 1 1 1
  spline S55 degree 3 poles (10.0655, -5.914) (9.9118, -5.7583) (9.8067, -5.6842) (9.771, -5.6609) knots 0 0 0 0 1 1 1 1
  line L28 (9.771, -5.6609) -> (9.5721, -5.5457)
  arc A29 (9.5721, -5.5457) -> (9.929, -4.8779) centre (0, 0) ccw
  line L29 (9.929, -4.8779) -> (10.1353, -4.9792)
  spline S56 degree 3 poles (10.1353, -4.9792) (10.1746, -4.996) (10.2945, -5.0423) (10.5094, -5.0835) knots 0 0 0 0 1 1 1 1
  spline S57 degree 3 poles (10.5094, -5.0835) (10.7664, -5.1326) (11.1523, -5.1719) (11.6708, -5.1356) knots 0 0 0 0 1 1 1 1
  arc A30 (11.6708, -5.1356) -> (11.8839, -4.6211) centre (0, 0) ccw
  spline S58 degree 3 poles (11.8839, -4.6211) (11.543, -4.2287) (11.2423, -3.9837) (11.0259, -3.8367) knots 0 0 0 0 1 1 1 1
  spline S59 degree 3 poles (11.0259, -3.8367) (10.8448, -3.7139) (10.7272, -3.6618) (10.6876, -3.6459) knots 0 0 0 0 1 1 1 1
  line L30 (10.6876, -3.6459) -> (10.47, -3.5717)
  arc A31 (10.47, -3.5717) -> (10.6899, -2.8471) centre (0, 0) ccw
  line L31 (10.6899, -2.8471) -> (10.912, -2.9063)
  spline S60 degree 3 poles (10.912, -2.9063) (10.9537, -2.915) (11.0804, -2.937) (11.2992, -2.9356) knots 0 0 0 0 1 1 1 1
  spline S61 degree 3 poles (11.2992, -2.9356) (11.5608, -2.9336) (11.947, -2.8969) (12.4485, -2.76) knots 0 0 0 0 1 1 1 1
  arc A32 (12.4485, -2.76) -> (12.5571, -2.2139) centre (0, 0) ccw
  spline S62 degree 3 poles (12.5571, -2.2139) (12.1462, -1.8956) (11.8034, -1.7139) (11.5625, -1.6119) knots 0 0 0 0 1 1 1 1
  spline S63 degree 3 poles (11.5625, -1.6119) (11.3609, -1.5268) (11.2354, -1.4987) (11.1935, -1.4908) knots 0 0 0 0 1 1 1 1
  line L32 (11.1935, -1.4908) -> (10.9657, -1.4605)
  arc A33 (10.9657, -1.4605) -> (11.0399, -0.7069) centre (0, 0) ccw
  line L33 (11.0399, -0.7069) -> (11.2693, -0.7216)
  spline S64 degree 3 poles (11.2693, -0.7216) (11.3119, -0.7221) (11.4405, -0.7189) (11.6548, -0.6748) knots 0 0 0 0 1 1 1 1
  spline S65 degree 3 poles (11.6548, -0.6748) (11.911, -0.6218) (12.2826, -0.5105) (12.7477, -0.2784) knots 0 0 0 0 1 1 1 1
  arc A34 (12.7477, -0.2784) -> (12.7477, 0.2784) centre (0, 0) ccw
  spline S66 degree 3 poles (12.7477, 0.2784) (12.2826, 0.5105) (11.911, 0.6218) (11.6548, 0.6748) knots 0 0 0 0 1 1 1 1
  spline S67 degree 3 poles (11.6548, 0.6748) (11.4405, 0.7189) (11.3119, 0.7221) (11.2693, 0.7216) knots 0 0 0 0 1 1 1 1
  line L34 (11.2693, 0.7216) -> (11.0399, 0.7069)
  arc A35 (11.0399, 0.7069) -> (10.9657, 1.4605) centre (0, 0) ccw
  line L35 (10.9657, 1.4605) -> (11.1935, 1.4908)
  spline S68 degree 3 poles (11.1935, 1.4908) (11.2354, 1.4987) (11.3609, 1.5268) (11.5625, 1.6119) knots 0 0 0 0 1 1 1 1
  spline S69 degree 3 poles (11.5625, 1.6119) (11.8034, 1.7139) (12.1462, 1.8956) (12.5571, 2.2139) knots 0 0 0 0 1 1 1 1
  arc A36 (12.5571, 2.2139) -> (12.4485, 2.76) centre (0, 0) ccw
  spline S70 degree 3 poles (12.4485, 2.76) (11.947, 2.8969) (11.5608, 2.9336) (11.2992, 2.9356) knots 0 0 0 0 1 1 1 1
  spline S71 degree 3 poles (11.2992, 2.9356) (11.0804, 2.937) (10.9537, 2.915) (10.912, 2.9063) knots 0 0 0 0 1 1 1 1
  line L36 (10.912, 2.9063) -> (10.6899, 2.8471)
  arc A37 (10.6899, 2.8471) -> (10.47, 3.5717) centre (0, 0) ccw
  line L37 (10.47, 3.5717) -> (10.6876, 3.6459)
  spline S72 degree 3 poles (10.6876, 3.6459) (10.7272, 3.6618) (10.8448, 3.7139) (11.0259, 3.8367) knots 0 0 0 0 1 1 1 1
  spline S73 degree 3 poles (11.0259, 3.8367) (11.2423, 3.9837) (11.543, 4.2287) (11.8839, 4.6211) knots 0 0 0 0 1 1 1 1
  arc A38 (11.8839, 4.6211) -> (11.6708, 5.1356) centre (0, 0) ccw
  spline S74 degree 3 poles (11.6708, 5.1356) (11.1523, 5.1719) (10.7664, 5.1326) (10.5094, 5.0835) knots 0 0 0 0 1 1 1 1
  spline S75 degree 3 poles (10.5094, 5.0835) (10.2945, 5.0423) (10.1746, 4.996) (10.1353, 4.9792) knots 0 0 0 0 1 1 1 1
  line L38 (10.1353, 4.9792) -> (9.929, 4.8779)
  arc A39 (9.929, 4.8779) -> (9.5721, 5.5457) centre (0, 0) ccw
  line L39 (9.5721, 5.5457) -> (9.771, 5.6609)
  spline S76 degree 3 poles (9.771, 5.6609) (9.8067, 5.6842) (9.9118, 5.7583) (10.0655, 5.914) knots 0 0 0 0 1 1 1 1
  spline S77 degree 3 poles (10.0655, 5.914) (10.2491, 6.1004) (10.4962, 6.3994) (10.754, 6.8508) knots 0 0 0 0 1 1 1 1
  arc A40 (10.754, 6.8508) -> (10.4447, 7.3137) centre (0, 0) ccw
  spline S78 degree 3 poles (10.4447, 7.3137) (9.929, 7.2483) (9.5582, 7.1344) (9.3157, 7.0361) knots 0 0 0 0 1 1 1 1
  spline S79 degree 3 poles (9.3157, 7.0361) (9.113, 6.9538) (9.0044, 6.8849) (8.9692, 6.8609) knots 0 0 0 0 1 1 1 1
  line L40 (8.9692, 6.8609) -> (8.7866, 6.7212)
  arc A41 (8.7866, 6.7212) -> (8.3062, 7.3065) centre (0, 0) ccw
  line L41 (8.3062, 7.3065) -> (8.4788, 7.4584)
  spline S80 degree 3 poles (8.4788, 7.4584) (8.5093, 7.4882) (8.598, 7.5813) (8.7184, 7.7641) knots 0 0 0 0 1 1 1 1
  spline S81 degree 3 poles (8.7184, 7.7641) (8.862, 7.9827) (9.046, 8.3242) (9.2109, 8.8171) knots 0 0 0 0 1 1 1 1
  arc A42 (9.2109, 8.8171) -> (8.8171, 9.2109) centre (0, 0) ccw
  spline S82 degree 3 poles (8.8171, 9.2109) (8.3242, 9.046) (7.9827, 8.862) (7.7641, 8.7184) knots 0 0 0 0 1 1 1 1
  spline S83 degree 3 poles (7.7641, 8.7184) (7.5813, 8.598) (7.4882, 8.5093) (7.4584, 8.4788) knots 0 0 0 0 1 1 1 1
  line L42 (7.4584, 8.4788) -> (7.3065, 8.3062)
  arc A43 (7.3065, 8.3062) -> (6.7212, 8.7866) centre (0, 0) ccw
  line L43 (6.7212, 8.7866) -> (6.8609, 8.9692)
  spline S84 degree 3 poles (6.8609, 8.9692) (6.8849, 9.0044) (6.9538, 9.113) (7.0361, 9.3157) knots 0 0 0 0 1 1 1 1
  spline S85 degree 3 poles (7.0361, 9.3157) (7.1344, 9.5582) (7.2483, 9.929) (7.3137, 10.4447) knots 0 0 0 0 1 1 1 1
  arc A44 (7.3137, 10.4447) -> (6.8508, 10.754) centre (0, 0) ccw
  spline S86 degree 3 poles (6.8508, 10.754) (6.3994, 10.4962) (6.1004, 10.2491) (5.914, 10.0655) knots 0 0 0 0 1 1 1 1
  spline S87 degree 3 poles (5.914, 10.0655) (5.7583, 9.9118) (5.6842, 9.8067) (5.6609, 9.771) knots 0 0 0 0 1 1 1 1
  line L44 (5.6609, 9.771) -> (5.5457, 9.5721)
  arc A45 (5.5457, 9.5721) -> (4.8779, 9.929) centre (0, 0) ccw
  line L45 (4.8779, 9.929) -> (4.9792, 10.1353)
  spline S88 degree 3 poles (4.9792, 10.1353) (4.996, 10.1746) (5.0423, 10.2945) (5.0835, 10.5094) knots 0 0 0 0 1 1 1 1
  spline S89 degree 3 poles (5.0835, 10.5094) (5.1326, 10.7664) (5.1719, 11.1523) (5.1356, 11.6708) knots 0 0 0 0 1 1 1 1
  arc A46 (5.1356, 11.6708) -> (4.6211, 11.8839) centre (0, 0) ccw
  spline S90 degree 3 poles (4.6211, 11.8839) (4.2287, 11.543) (3.9837, 11.2423) (3.8367, 11.0259) knots 0 0 0 0 1 1 1 1
  spline S91 degree 3 poles (3.8367, 11.0259) (3.7139, 10.8448) (3.6618, 10.7272) (3.6459, 10.6876) knots 0 0 0 0 1 1 1 1
  line L46 (3.6459, 10.6876) -> (3.5717, 10.47)
  arc A47 (3.5717, 10.47) -> (2.8471, 10.6899) centre (0, 0) ccw
  line L47 (2.8471, 10.6899) -> (2.9063, 10.912)
  spline S92 degree 3 poles (2.9063, 10.912) (2.915, 10.9537) (2.937, 11.0804) (2.9356, 11.2992) knots 0 0 0 0 1 1 1 1
  spline S93 degree 3 poles (2.9356, 11.2992) (2.9336, 11.5608) (2.8969, 11.947) (2.76, 12.4485) knots 0 0 0 0 1 1 1 1
  arc A48 (2.76, 12.4485) -> (2.2139, 12.5571) centre (0, 0) ccw
  spline S94 degree 3 poles (2.2139, 12.5571) (1.8956, 12.1462) (1.7139, 11.8034) (1.6119, 11.5625) knots 0 0 0 0 1 1 1 1
  spline S95 degree 3 poles (1.6119, 11.5625) (1.5268, 11.3609) (1.4987, 11.2354) (1.4908, 11.1935) knots 0 0 0 0 1 1 1 1
  line L48 (1.4908, 11.1935) -> (1.4605, 10.9657)
  arc A49 (1.4605, 10.9657) -> (0.7069, 11.0399) centre (0, 0) ccw
  line L49 (0.7069, 11.0399) -> (0.7216, 11.2693)
  spline S96 degree 3 poles (0.7216, 11.2693) (0.7221, 11.3119) (0.7189, 11.4405) (0.6748, 11.6548) knots 0 0 0 0 1 1 1 1
  spline S97 degree 3 poles (0.6748, 11.6548) (0.6218, 11.911) (0.5105, 12.2826) (0.2784, 12.7477) knots 0 0 0 0 1 1 1 1
  arc A50 (0.2784, 12.7477) -> (-0.2784, 12.7477) centre (0, 0) ccw
  spline S98 degree 3 poles (-0.2784, 12.7477) (-0.5105, 12.2826) (-0.6218, 11.911) (-0.6748, 11.6548) knots 0 0 0 0 1 1 1 1
  spline S99 degree 3 poles (-0.6748, 11.6548) (-0.7189, 11.4405) (-0.7221, 11.3119) (-0.7216, 11.2693) knots 0 0 0 0 1 1 1 1
  line L50 (-0.7216, 11.2693) -> (-0.7069, 11.0399)
  arc A51 (-0.7069, 11.0399) -> (-1.4605, 10.9657) centre (0, 0) ccw
  line L51 (-1.4605, 10.9657) -> (-1.4908, 11.1935)
  spline S100 degree 3 poles (-1.4908, 11.1935) (-1.4987, 11.2354) (-1.5268, 11.3609) (-1.6119, 11.5625) knots 0 0 0 0 1 1 1 1
  spline S101 degree 3 poles (-1.6119, 11.5625) (-1.7139, 11.8034) (-1.8956, 12.1462) (-2.2139, 12.5571) knots 0 0 0 0 1 1 1 1
  arc A52 (-2.2139, 12.5571) -> (-2.76, 12.4485) centre (0, 0) ccw
  spline S102 degree 3 poles (-2.76, 12.4485) (-2.8969, 11.947) (-2.9336, 11.5608) (-2.9356, 11.2992) knots 0 0 0 0 1 1 1 1
  spline S103 degree 3 poles (-2.9356, 11.2992) (-2.937, 11.0804) (-2.915, 10.9537) (-2.9063, 10.912) knots 0 0 0 0 1 1 1 1
  line L52 (-2.9063, 10.912) -> (-2.8471, 10.6899)
  arc A53 (-2.8471, 10.6899) -> (-3.5717, 10.47) centre (0, 0) ccw
  line L53 (-3.5717, 10.47) -> (-3.6459, 10.6876)
  spline S104 degree 3 poles (-3.6459, 10.6876) (-3.6618, 10.7272) (-3.7139, 10.8448) (-3.8367, 11.0259) knots 0 0 0 0 1 1 1 1
  spline S105 degree 3 poles (-3.8367, 11.0259) (-3.9837, 11.2423) (-4.2287, 11.543) (-4.6211, 11.8839) knots 0 0 0 0 1 1 1 1
  arc A54 (-4.6211, 11.8839) -> (-5.1356, 11.6708) centre (0, 0) ccw
  spline S106 degree 3 poles (-5.1356, 11.6708) (-5.1719, 11.1523) (-5.1326, 10.7664) (-5.0835, 10.5094) knots 0 0 0 0 1 1 1 1
  spline S107 degree 3 poles (-5.0835, 10.5094) (-5.0423, 10.2945) (-4.996, 10.1746) (-4.9792, 10.1353) knots 0 0 0 0 1 1 1 1
  line L54 (-4.9792, 10.1353) -> (-4.8779, 9.929)
  arc A55 (-4.8779, 9.929) -> (-5.5457, 9.5721) centre (0, 0) ccw
  line L55 (-5.5457, 9.5721) -> (-5.6609, 9.771)
  spline S108 degree 3 poles (-5.6609, 9.771) (-5.6842, 9.8067) (-5.7583, 9.9118) (-5.914, 10.0655) knots 0 0 0 0 1 1 1 1
  spline S109 degree 3 poles (-5.914, 10.0655) (-6.1004, 10.2491) (-6.3994, 10.4962) (-6.8508, 10.754) knots 0 0 0 0 1 1 1 1
  arc A56 (-6.8508, 10.754) -> (-7.3137, 10.4447) centre (0, 0) ccw
  spline S110 degree 3 poles (-7.3137, 10.4447) (-7.2483, 9.929) (-7.1344, 9.5582) (-7.0361, 9.3157) knots 0 0 0 0 1 1 1 1
  spline S111 degree 3 poles (-7.0361, 9.3157) (-6.9538, 9.113) (-6.8849, 9.0044) (-6.8609, 8.9692) knots 0 0 0 0 1 1 1 1
  line L56 (-6.8609, 8.9692) -> (-6.7212, 8.7866)
  arc A57 (-6.7212, 8.7866) -> (-7.3065, 8.3062) centre (0, 0) ccw
  line L57 (-7.3065, 8.3062) -> (-7.4584, 8.4788)
  spline S112 degree 3 poles (-7.4584, 8.4788) (-7.4882, 8.5093) (-7.5813, 8.598) (-7.7641, 8.7184) knots 0 0 0 0 1 1 1 1
  spline S113 degree 3 poles (-7.7641, 8.7184) (-7.9827, 8.862) (-8.3242, 9.046) (-8.8171, 9.2109) knots 0 0 0 0 1 1 1 1
  arc A58 (-8.8171, 9.2109) -> (-9.2109, 8.8171) centre (0, 0) ccw
  spline S114 degree 3 poles (-9.2109, 8.8171) (-9.046, 8.3242) (-8.862, 7.9827) (-8.7184, 7.7641) knots 0 0 0 0 1 1 1 1
  spline S115 degree 3 poles (-8.7184, 7.7641) (-8.598, 7.5813) (-8.5093, 7.4882) (-8.4788, 7.4584) knots 0 0 0 0 1 1 1 1
  line L58 (-8.4788, 7.4584) -> (-8.3062, 7.3065)
  arc A59 (-8.3062, 7.3065) -> (-8.7866, 6.7212) centre (0, 0) ccw
  line L59 (-8.7866, 6.7212) -> (-8.9692, 6.8609)
  spline S116 degree 3 poles (-8.9692, 6.8609) (-9.0044, 6.8849) (-9.113, 6.9538) (-9.3157, 7.0361) knots 0 0 0 0 1 1 1 1
  spline S117 degree 3 poles (-9.3157, 7.0361) (-9.5582, 7.1344) (-9.929, 7.2483) (-10.4447, 7.3137) knots 0 0 0 0 1 1 1 1
  arc A60 (-10.4447, 7.3137) -> (-10.754, 6.8508) centre (0, 0) ccw
  spline S118 degree 3 poles (-10.754, 6.8508) (-10.4962, 6.3994) (-10.2491, 6.1004) (-10.0655, 5.914) knots 0 0 0 0 1 1 1 1
  spline S119 degree 3 poles (-10.0655, 5.914) (-9.9118, 5.7583) (-9.8067, 5.6842) (-9.771, 5.6609) knots 0 0 0 0 1 1 1 1
  line L60 (-9.771, 5.6609) -> (-9.5721, 5.5457)
  arc A61 (-9.5721, 5.5457) -> (-9.929, 4.8779) centre (0, 0) ccw
  line L61 (-9.929, 4.8779) -> (-10.1353, 4.9792)
  spline S120 degree 3 poles (-10.1353, 4.9792) (-10.1746, 4.996) (-10.2945, 5.0423) (-10.5094, 5.0835) knots 0 0 0 0 1 1 1 1
  spline S121 degree 3 poles (-10.5094, 5.0835) (-10.7664, 5.1326) (-11.1523, 5.1719) (-11.6708, 5.1356) knots 0 0 0 0 1 1 1 1
  arc A62 (-11.6708, 5.1356) -> (-11.8839, 4.6211) centre (0, 0) ccw
  spline S122 degree 3 poles (-11.8839, 4.6211) (-11.543, 4.2287) (-11.2423, 3.9837) (-11.0259, 3.8367) knots 0 0 0 0 1 1 1 1
  spline S123 degree 3 poles (-11.0259, 3.8367) (-10.8448, 3.7139) (-10.7272, 3.6618) (-10.6876, 3.6459) knots 0 0 0 0 1 1 1 1
  line L62 (-10.6876, 3.6459) -> (-10.47, 3.5717)
  arc A63 (-10.47, 3.5717) -> (-10.6899, 2.8471) centre (0, 0) ccw
  line L63 (-10.6899, 2.8471) -> (-10.912, 2.9063)
  spline S124 degree 3 poles (-10.912, 2.9063) (-10.9537, 2.915) (-11.0804, 2.937) (-11.2992, 2.9356) knots 0 0 0 0 1 1 1 1
  spline S125 degree 3 poles (-11.2992, 2.9356) (-11.5608, 2.9336) (-11.947, 2.8969) (-12.4485, 2.76) knots 0 0 0 0 1 1 1 1
  arc A64 (-12.4485, 2.76) -> (-12.5571, 2.2139) centre (0, 0) ccw
  spline S126 degree 3 poles (-12.5571, 2.2139) (-12.1462, 1.8956) (-11.8034, 1.7139) (-11.5625, 1.6119) knots 0 0 0 0 1 1 1 1
  spline S127 degree 3 poles (-11.5625, 1.6119) (-11.3609, 1.5268) (-11.2354, 1.4987) (-11.1935, 1.4908) knots 0 0 0 0 1 1 1 1
  circle A65 centre (0, 0) radius 3.75
  dimension "d3" = 7.5
  constraint concentric A5 A65
  measures "d3" diameter of A65
extrude "Extrude2" add sketch "Sketch1 (2)" against normal blind 25 contours A0 A65 in component "Spur Gear (32 teeth)"
extrude "Extrude3" add sketch "Sketch1 (2)" against normal blind 40 contours A0 A65 in component "Spur Gear (32 teeth)"
extrude "Extrude4" add sketch "Sketch1 (2)" along normal blind 15 contours A0 A65 in component "Spur Gear (32 teeth)"
sketch "Sketch2 (2)" plane through (0, 40, 0) normal (0, 1, 0) x (-1, 0, 0)
  circle A0 centre (0, 0) radius 3.75
extrude "Extrude5" cut sketch "Sketch2 (2)" against normal blind 1 in component "Spur Gear (32 teeth)"
sketch "Sketch3" plane through (0, 39, 0) normal (0, 1, 0) x (-1, 0, 0)
  circle A0 centre (0, 0) radius 3.75
  circle A1 centre (0, 0) radius 2
  dimension "d13" = 4
  constraint concentric A0 A1
  measures "d13" diameter of A1
extrude "Extrude6" cut sketch "Sketch3" against normal blind 5 contours A1 in component "Spur Gear (32 teeth)"
extrude "Extrude7" add 1 faces at (-3.1527, 39, -0.1863) along direction (0, 1, 0) blind 1 in component "Spur Gear (32 teeth)"
extrude "Extrude8" cut 1 faces at (1.1262, -15, 0.5424) along direction (0, 1, 0) blind 1 in component "Spur Gear (32 teeth)"
thread "Thread1" "ISO Metric profile 4.0 M4x0.7 6H" major diameter 4.1095 minor diameter 3.332 pitch 0.7 angle 60 modelled right hand crest width 0.193 on face at (-1.9975, 38, -0.0997) crest through (-1.666, 39.825, 0) in component "Spur Gear (32 teeth)"
component "Spur Gear (32 teeth)" placed x (1, 0, 0) y (0, 1, 0) z (0, 0, 1) at (0, 0, 0)
